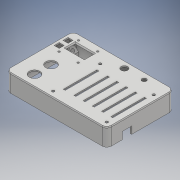
# Autodesk Inventor part: TestingRemoteHousing
Saved by Autodesk Inventor 2018.3 (Build 223284000, 284)
## iProperties
Created: 2019-03-25
Part Number: TestingRemoteHousing
Material: Generic
Document SubType Name: Modeling
Designer: matth
Density: 1 g/cm^3
Appearance: Default
Author: matth
Autodesk Inventor part; units mm, degrees
ref_plane "YZ Plane" through (0, 0, 0) normal (1, 0, 0) x (0, 1, 0)
ref_plane "XZ Plane" through (0, 0, 0) normal (0, 1, 0) x (-1, 0, 0)
ref_plane "XY Plane" through (0, 0, 0) normal (0, 0, 1) x (1, 0, 0)
sketch "Sketch1" plane through (0, 0, 0) normal (0, 0, 1) x (1, 0, 0)
  line L0 (-6.9712, 4.0639) -> (131.4288, 4.0639)
  line L1 (138.4288, -2.9361) -> (138.4288, -90.5361)
  line L2 (131.4288, -97.5361) -> (-6.9712, -97.5361)
  line L3 (-13.9712, -90.5361) -> (-13.9712, -2.9361)
  arc A0 (-6.9712, 4.0639) -> (-13.9712, -2.9361) centre (-6.9712, -2.9361) ccw
  arc A1 (-13.9712, -90.5361) -> (-6.9712, -97.5361) centre (-6.9712, -90.5361) ccw
  arc A2 (131.4288, -97.5361) -> (138.4288, -90.5361) centre (131.4288, -90.5361) ccw
  arc A3 (138.4288, -2.9361) -> (131.4288, 4.0639) centre (131.4288, -2.9361) ccw
  circle A4 centre (103.4288, -5.9361) radius 3.43
  circle A5 centre (130.4288, -89.5361) radius 2
  circle A6 centre (49.2288, -89.5361) radius 2
  circle A7 centre (49.2288, -18.3361) radius 2
  circle A8 centre (130.4288, -18.3361) radius 2
  circle A9 centre (2.0288, -3.9361) radius 1.5
  circle A10 centre (30.9848, -3.9361) radius 1.5
  circle A11 centre (2.0288, -33.4001) radius 1.5
  circle A12 centre (30.9848, -33.4001) radius 1.5
  circle A13 centre (13.0288, -56.5361) radius 8
  circle A14 centre (13.0288, -81.5361) radius 8
  line L4 (-9.7712, -7.9361) -> (-2.0712, -7.9361)
  line L5 (-2.0712, -7.9361) -> (-2.0712, -15.6361)
  line L6 (-2.0712, -15.6361) -> (-9.7712, -15.6361)
  line L7 (-9.7712, -15.6361) -> (-9.7712, -7.9361)
  line L8 (-9.7712, -21.3361) -> (-2.0712, -21.3361)
  line L9 (-2.0712, -21.3361) -> (-2.0712, -29.0361)
  line L10 (-2.0712, -29.0361) -> (-9.7712, -29.0361)
  line L11 (-9.7712, -29.0361) -> (-9.7712, -21.3361)
  circle A15 centre (73.4288, -5.9361) radius 5
  line L12 (2.0288, -24.0021) -> (30.9848, -24.0021)
  line L13 (30.9848, -24.0021) -> (30.9848, -9.0021)
  line L14 (30.9848, -9.0021) -> (2.0288, -9.0021)
  line L15 (2.0288, -9.0021) -> (2.0288, -24.0021)
  line L16 (54.5635, -28.5361) -> (57.5635, -28.5361)
  line L17 (57.5635, -28.5361) -> (57.5635, -79.5361)
  line L18 (57.5635, -79.5361) -> (54.5635, -79.5361)
  line L19 (54.5635, -79.5361) -> (54.5635, -28.5361)
  line L20 (70.5888, -79.5361) -> (73.5888, -79.5361)
  line L21 (73.5888, -79.5361) -> (73.5888, -28.5361)
  line L22 (73.5888, -28.5361) -> (70.5888, -28.5361)
  line L23 (70.5888, -28.5361) -> (70.5888, -79.5361)
  line L24 (84.5588, -28.5361) -> (87.5588, -28.5361)
  line L25 (87.5588, -28.5361) -> (87.5588, -79.5361)
  line L26 (87.5588, -79.5361) -> (84.5588, -79.5361)
  line L27 (84.5588, -79.5361) -> (84.5588, -28.5361)
  line L28 (98.5288, -28.5361) -> (101.5288, -28.5361)
  line L29 (101.5288, -28.5361) -> (101.5288, -79.5361)
  line L30 (101.5288, -79.5361) -> (98.5288, -79.5361)
  line L31 (98.5288, -79.5361) -> (98.5288, -28.5361)
  line L32 (112.4288, -28.5361) -> (115.4288, -28.5361)
  line L33 (115.4288, -28.5361) -> (115.4288, -79.5361)
  line L34 (115.4288, -79.5361) -> (112.4288, -79.5361)
  line L35 (112.4288, -79.5361) -> (112.4288, -28.5361)
  line L36 (126.4688, -28.5361) -> (129.4688, -28.5361)
  line L37 (129.4688, -28.5361) -> (129.4688, -79.5361)
  line L38 (129.4688, -79.5361) -> (126.4688, -79.5361)
  line L39 (126.4688, -79.5361) -> (126.4688, -28.5361)
  point P0 (0, 0)
  point P1 (138.4288, -97.5361)
  point P2 (138.4288, 4.0639)
  point P3 (-13.9712, -97.5361)
  dimension "d0" = 152.4
  dimension "d1" = 101.6
  dimension "d2" = 7
  dimension "d3" = 6.86
  dimension "d4" = 10
  dimension "d5" = 35
  dimension "d6" = 4
  dimension "d7" = 4
  dimension "d8" = 4
  dimension "d9" = 81.2
  dimension "d10" = 8
  dimension "d11" = 0
  dimension "d12" = 71.2
  dimension "d13" = 4
  dimension "d14" = 8
  dimension "d15" = 3
  dimension "d16" = 3
  dimension "d17" = 28.956
  dimension "d18" = 16
  dimension "d19" = 3
  dimension "d20" = 29.464
  dimension "d21" = 3
  dimension "d22" = 16
  dimension "d23" = 16
  dimension "d24" = 16
  dimension "d25" = 63.2
  dimension "d26" = 27
  dimension "d27" = 27
  dimension "d28" = 25
  dimension "d29" = 8
  dimension "d30" = 0
  dimension "d31" = 7.7
  dimension "d32" = 7.7
  dimension "d33" = 4.2
  dimension "d34" = 12
  dimension "d35" = 7.7
  dimension "d36" = 10
  dimension "d37" = 10
  dimension "d38" = 65
  dimension "d39" = 0
  dimension "d40" = 28.956
  dimension "d41" = 15
  dimension "d42" = 9.398
  dimension "d43" = 0
  dimension "d44" = 3
  dimension "d45" = 51
  dimension "d46" = 10.2
  dimension "d47" = 3
  dimension "d48" = 51
  dimension "d49" = 3
  dimension "d50" = 51
  dimension "d51" = 3
  dimension "d52" = 51
  dimension "d53" = 3
  dimension "d54" = 51
  dimension "d55" = 3
  dimension "d56" = 51
  dimension "d57" = 21.36
  dimension "d58" = 35.33
  dimension "d59" = 49.3
  dimension "d60" = 63.2
  dimension "d61" = 80.24
  constraints: 80 end point, 20 parallel, 16 centre point, 10 horizontal, 10 perpendicular, 10 point on line, 8 point on circle, 8 tangent, 3 equal radius
  measures "d0" distance of point (138.429, -97.536) point (-13.971, -97.536)
  measures "d1" distance of point (138.429, 4.064) point (138.429, -97.536)
  measures "d2" radius of A0
  measures "d3" diameter of A4
  measures "d4" distance from line of L0 A4.centre
  measures "d5" distance from line of L1 A4.centre
  measures "d6" diameter of A5
  measures "d7" diameter of A6
  measures "d8" diameter of A7
  measures "d9" distance of A6.centre A5.centre
  measures "d10" distance from line of L1 A5.centre
  measures "d11" horizontal distance of A7.centre A6.centre
  measures "d12" distance of A6.centre A7.centre
  measures "d13" diameter of A8
  measures "d14" distance from line of L2 A5.centre
  measures "d15" diameter of A9
  measures "d16" diameter of A10
  measures "d17" distance of A10.centre A9.centre
  measures "d18" distance from line of L3 A9.centre
  measures "d19" diameter of A11
  measures "d20" distance of A9.centre A11.centre
  measures "d21" diameter of A12
  measures "d22" diameter of A13
  measures "d23" diameter of A14
  measures "d24" distance from line of L2 A14.centre
  measures "d25" distance from line of A6.centre L3
  measures "d26" distance from line of L3 A14.centre
  measures "d27" distance from line of A13.centre L3
  measures "d28" distance of A14.centre A13.centre
  measures "d29" distance from line of L0 A9.centre
  measures "d30" vertical distance of A11.centre A12.centre
  measures "d31" distance of L5.end L6.end
  measures "d32" distance of L4.end L5.end
  measures "d33" distance between parallel lines of L3 L7
  measures "d34" distance between parallel lines of L0 L4
  measures "d35" distance of L8.end L9.end
  measures "d36" diameter of A15
  measures "d37" distance from line of A15.centre L0
  measures "d38" distance from line of L1 A15.centre
  measures "d39" vertical distance of A8.centre A7.centre
  measures "d40" distance of L14.end L13.end
  measures "d41" distance of L12.end L13.end
  measures "d42" distance from line of L12 A11.centre
  measures "d43" distance from line of A10.centre L13
  measures "d44" distance of L17.end L18.end
  measures "d45" distance of L16.end L17.end
  measures "d46" distance from line of A7.centre L16
  measures "d47" distance of L22.end L21.end
  measures "d48" distance of L21.end L20.end
  measures "d49" distance of L25.end L26.end
  measures "d50" distance of L24.end L25.end
  measures "d51" distance of L29.end L30.end
  measures "d52" distance of L28.end L29.end
  measures "d53" distance of L33.end L34.end
  measures "d54" distance of L32.end L33.end
  measures "d55" distance of L37.end L38.end
  measures "d56" distance of L36.end L37.end
  measures "d57" distance from line of L23 A7.centre
  measures "d58" distance from line of A7.centre L27
  measures "d59" distance from line of L31 A7.centre
  measures "d60" distance from line of A7.centre L35
  measures "d61" distance from line of A7.centre L37
extrude "Extrusion1" add sketch "Sketch1" along normal blind 2
chamfer "Chamfer1" distance 1 distance2 2 1 edges at (30.9848, -16.5021, 2) measured on face at (31.4848, -16.5021, 2)
chamfer "Chamfer2" distance 1 distance2 2 2 edges at (31.4848, -9.0021, 2) (16.5068, -9.0021, 2) measured on face at (31.4848, -8.5021, 2) measured on face at (16.5068, -8.5021, 2)
chamfer "Chamfer3" distance 1 distance2 2 2 edges at (2.0288, -8.5021, 2) (2.0288, -16.5021, 2) measured on face at (1.5288, -8.5021, 2) measured on face at (1.5288, -16.5021, 2)
chamfer "Chamfer4" distance 1 distance2 2 3 edges at (1.5289, -24.0021, 2) (16.5068, -24.0021, 2) (31.4848, -24.0021, 2) measured on face at (31.4848, -24.5021, 2) measured on face at (1.5289, -24.5021, 2) measured on face at (16.5068, -24.5021, 2)
chamfer "Chamfer5" distance 0.5 distance2 2 8 edges at (-13.9712, -46.7361, 2) (-11.9209, -95.4858, 2) (62.2288, -97.5361, 2) (136.3786, -95.4858, 2) (138.4288, -46.7361, 2) (136.3786, 2.0136, 2) (62.2288, 4.0639, 2) (-11.9209, 2.0136, 2) measured on face at (136.025, 1.6601, 2) measured on face at (62.2288, -97.0361, 2) measured on face at (62.2288, 3.5639, 2) measured on face at (-11.5674, -95.1323, 2) measured on face at (-11.5674, 1.6601, 2) measured on face at (137.9288, -46.7361, 2) measured on face at (136.025, -95.1323, 2) measured on face at (-13.4712, -46.7361, 2)
sketch "Sketch2" plane through (0, 0, 0) normal (0, 0, -1) x (-1, 0, 0)
  line L0 (6.9712, -97.5361) -> (-131.4288, -97.5361) projected
  arc A0 (6.9712, -97.5361) -> (13.9712, -90.5361) centre (6.9712, -90.5361) ccw projected
  line L1 (13.9712, -2.9361) -> (13.9712, -90.5361) projected
  arc A1 (13.9712, -2.9361) -> (6.9712, 4.0639) centre (6.9712, -2.9361) ccw projected
  line L2 (-131.4288, 4.0639) -> (6.9712, 4.0639) projected
  arc A2 (-131.4288, 4.0639) -> (-138.4288, -2.9361) centre (-131.4288, -2.9361) ccw projected
  line L3 (-138.4288, -90.5361) -> (-138.4288, -2.9361) projected
  arc A3 (-138.4288, -90.5361) -> (-131.4288, -97.5361) centre (-131.4288, -90.5361) ccw projected
  line L4 (-131.4288, -95.5361) -> (6.9712, -95.5361)
  arc A4 (6.9712, -95.5361) -> (11.9712, -90.5361) centre (6.9712, -90.5361) ccw
  line L5 (11.9712, -90.5361) -> (11.9712, -2.9361)
  arc A5 (11.9712, -2.9361) -> (6.9712, 2.0639) centre (6.9712, -2.9361) ccw
  line L6 (6.9712, 2.0639) -> (-131.4288, 2.0639)
  arc A6 (-131.4288, 2.0639) -> (-136.4288, -2.9361) centre (-131.4288, -2.9361) ccw
  line L7 (-136.4288, -2.9361) -> (-136.4288, -90.5361)
  arc A7 (-136.4288, -90.5361) -> (-131.4288, -95.5361) centre (-131.4288, -90.5361) ccw
  point P0 (0, 0)
  dimension "d79" = 2
  constraints: 8 end point, 8 point on circle, 4 centre point, 7 other
  measures "d79" distance between parallel lines of L0 L4
extrude "Extrusion2" add sketch "Sketch2" along normal blind 25
sketch "Sketch3" plane through (0, 0, -25) normal (0, 0, -1) x (-1, 0, 0)
  line L0 (-131.4288, 2.0639) -> (6.9712, 2.0639) projected
  arc A0 (-131.4288, 2.0639) -> (-136.4288, -2.9361) centre (-131.4288, -2.9361) ccw projected
  line L1 (-136.4288, -90.5361) -> (-136.4288, -2.9361) projected
  arc A1 (-136.4288, -90.5361) -> (-131.4288, -95.5361) centre (-131.4288, -90.5361) ccw projected
  line L2 (6.9712, -95.5361) -> (-131.4288, -95.5361) projected
  arc A2 (6.9712, -95.5361) -> (11.9712, -90.5361) centre (6.9712, -90.5361) ccw projected
  line L3 (11.9712, -2.9361) -> (11.9712, -90.5361) projected
  arc A3 (11.9712, -2.9361) -> (6.9712, 2.0639) centre (6.9712, -2.9361) ccw projected
  line L4 (3.9712, -5.9361) -> (-128.4288, -5.9361)
  line L5 (-128.4288, -5.9361) -> (-128.4288, -87.5361)
  line L6 (-128.4288, -87.5361) -> (3.9712, -87.5361)
  line L7 (3.9712, -87.5361) -> (3.9712, -5.9361)
  line L8 (-128.4288, -5.9361) -> (-128.4288, 2.0639)
  line L9 (-128.4288, -5.9361) -> (-136.4288, -5.9361)
  line L10 (3.9712, -5.9361) -> (3.9712, 2.0639)
  line L11 (3.9712, -5.9361) -> (11.9712, -5.9361)
  line L12 (-128.4288, -87.5361) -> (11.9712, -87.5361)
  line L13 (11.9712, -90.5361) -> (11.9712, -2.9361) projected
  line L14 (3.9712, -5.9361) -> (3.9712, -95.5361)
  line L15 (-131.4288, -95.5361) -> (6.9712, -95.5361) projected
  line L16 (-128.4288, -87.5361) -> (-136.4288, -87.5361)
  line L17 (-136.4288, -2.9361) -> (-136.4288, -90.5361) projected
  line L18 (-128.4288, -87.5361) -> (-128.4288, -95.5361)
  point P0 (0, 0)
  dimension "d82" = 8
  constraints: 24 end point, 12 point on line, 4 perpendicular, 2 vertical, 3 other
  measures "d82" distance between parallel lines of L0 L4
extrude "Extrusion3" add sketch "Sketch3" against normal blind 14 contours L0 L8 L9 L1 A0 | L0 A3 L3 L11 L10 | L11 L3 L12 L7 | L18 L2 A1 L1 L16 | L12 L3 A2 L2 L14
chamfer "Chamfer6" distance 8 angle 45 3 edges at (128.4288, -91.5361, -11) (128.4288, -1.9361, -11) (-3.9712, -46.7361, -11)
sketch "Sketch4" plane through (0, 0, -25) normal (0, 0, -1) x (-1, 0, 0)
  circle A0 centre (-131.4288, -90.5361) radius 1.75
  line L0 (-138.4288, -2.9361) -> (-138.4288, -90.5361) projected
  line L1 (-131.4288, -97.5361) -> (6.9712, -97.5361) projected
  circle A1 centre (-131.4288, -2.9361) radius 1.75
  line L2 (6.9712, 4.0639) -> (-131.4288, 4.0639) projected
  circle A2 centre (6.9712, -2.9361) radius 1.75
  line L3 (13.9712, -90.5361) -> (13.9712, -2.9361) projected
  circle A3 centre (6.9712, -90.5361) radius 1.75
  point P0 (0, 0)
  dimension "d88" = 3.5
  dimension "d89" = 7
  dimension "d90" = 7
  dimension "d91" = 3.5
  dimension "d92" = 7
  dimension "d93" = 7
  dimension "d94" = 3.5
  dimension "d95" = 7
  dimension "d96" = 7
  dimension "d97" = 3.5
  dimension "d98" = 7
  dimension "d99" = 7
  constraints: 4 centre point
  measures "d88" diameter of A0
  measures "d89" distance from line of L0 A0.centre
  measures "d90" distance from line of L1 A0.centre
  measures "d91" diameter of A1
  measures "d92" distance from line of L0 A1.centre
  measures "d93" distance from line of L2 A1.centre
  measures "d94" diameter of A2
  measures "d95" distance from line of L3 A2.centre
  measures "d96" distance from line of L2 A2.centre
  measures "d97" diameter of A3
  measures "d98" distance from line of L1 A3.centre
  measures "d99" distance from line of L3 A3.centre
extrude "Extrusion4" cut sketch "Sketch4" against normal blind 12
sketch "Sketch5" plane through (138.4288, -90.5361, 0) normal (1, 0, 0) x (0, 0, -1)
  line L0 (-2, -1) -> (-2, 3) projected
  line L1 (-2, 70.2) -> (-2, 74.2) projected
  line L2 (14, 16.5909) -> (25, 16.5909)
  line L3 (25, 16.5909) -> (25, 30.5909)
  line L4 (25, 30.5909) -> (14, 30.5909)
  line L5 (14, 30.5909) -> (14, 16.5909)
  line L6 (-2, 87.6) -> (-2, 0) projected
  line L7 (25, 87.6) -> (25, 0) projected
  point P0 (0, 90.5361)
  point P1 (-2, 1)
  point P2 (-2, 72.2)
  dimension "d102" = 11
  dimension "d103" = 14
  dimension "d105" = 0
  constraints: 8 end point, 2 midpoint, 2 parallel, 1 horizontal, 1 perpendicular
  measures "d102" distance of L4.end L3.end
  measures "d103" distance of L3.end L2.end
  measures "d105" distance between parallel lines of L7 L3
extrude "Extrusion5" cut sketch "Sketch5" against normal blind 10
sketch "Sketch6" plane through (0, 0, -25) normal (0, 0, -1) x (-1, 0, 0)
  line L0 (3.9712, 2.0639) -> (3.9712, -95.5361) projected
  line L1 (13.9712, -90.5361) -> (13.9712, -2.9361) projected
  line L2 (3.9712, -87.5361) -> (11.9712, -87.5361)
  line L3 (11.9712, -90.5361) -> (11.9712, -2.9361) projected
  line L4 (11.9712, -5.9361) -> (3.9712, -5.9361)
  line L5 (-128.4288, -87.5361) -> (-136.4288, -87.5361) projected
  line L6 (-136.4288, -5.9361) -> (-128.4288, -5.9361) projected
  line L7 (3.9712, -87.5361) -> (3.9712, -5.9361)
  line L8 (11.9712, -5.9361) -> (11.9712, -87.5361)
  point P0 (0, 0)
  dimension "d108" = 0
  dimension "d109" = 0
  constraints: 8 end point, 3 point on line, 1 collinear, 1 horizontal, 1 perpendicular, 1 vertical
  measures "d108" distance between parallel lines of L5 L2
  measures "d109" distance between parallel lines of L6 L4
extrude "Extrusion6" cut sketch "Sketch6" against normal up to surface (25 mm away)
equation "\"d27\" = d26"
body "Solid1"
